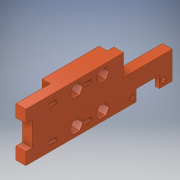
# Autodesk Inventor part: carriage Cartridge adapter
Saved by Autodesk Inventor 2018 (Build 220112000, 112)
## iProperties
Created: 2013-09-29
Part Number: carriage Cartridge adapter
Material: ABS Plastic
Document SubType Name: Modeling
Designer: Gabriel Smolnycki
Mass: 15.6927 g
Surface Area: 77.7092 cm^2
Volume: 14.8045 cm^3
Density: 1.06 g/cm^3
Appearance: Smooth - Light Orange
Author: Gabriel Smolnycki
Sending System: SolidWorks 2017
Last Author: Gabriel Smolnycki
Last Saved: 2017-09-14
Autodesk Inventor part; units mm, degrees
ref_plane "Work Plane1" through (0, 30, 0) normal (0, 1, 0) x (-1, 0, 0)
sketch "Sketch1" plane through (0, 30, 0) normal (0, 1, 0) x (-1, 0, 0)
  line L0 (-11, 41) -> (-11, -48.8)
  line L1 (0, -15) -> (-5, -15)
  line L2 (0, -15) -> (0, 41)
  line L3 (0, 41) -> (-11, 41)
  line L4 (-11, -48.8) -> (-5, -48.8)
  line L5 (-5, -48.8) -> (-5, -15)
  constraints: 12 end point, 3 horizontal, 3 vertical
extrude "Extrusion16" add sketch "Sketch1" against normal blind 30
ref_plane "Work Plane2" through (0, 0, -40.8) normal (0, 0, 1) x (1, 0, 0)
sketch "Sketch2" plane through (0, 0, -40.8) normal (0, 0, 1) x (1, 0, 0)
  line L0 (5, 7) -> (11, 7)
  line L1 (5, 0) -> (5, 7)
  line L2 (11, 0) -> (11, 7)
  line L3 (11, 0) -> (5, 0)
  constraints: 8 end point, 2 horizontal, 2 vertical
extrude "Extrusion15" cut sketch "Sketch2" along normal blind 14
sketch "Sketch3" plane through (11, 30, 41) normal (1, 0, 0) x (0, 0, -1)
  line L0 (40.5, -4) -> (35.5, -4)
  line L1 (40.5, -26) -> (40.5, -4)
  line L2 (35.5, -4) -> (35.5, -26)
  line L3 (35.5, -26) -> (40.5, -26)
  constraints: 8 end point, 2 horizontal, 2 vertical
extrude "Extrusion14" cut sketch "Sketch3" against normal blind 11
ref_plane "Work Plane3" through (0, 21, 0) normal (0, 1, 0) x (-1, 0, 0)
sketch "Sketch4" plane through (0, 21, 0) normal (0, 1, 0) x (-1, 0, 0)
  line L0 (0, 41) -> (-2, 41)
  line L1 (0, 5.5) -> (0, 41)
  line L2 (0, 5.5) -> (-2, 5.5)
  line L3 (-2, 5.5) -> (-2, 41)
  constraints: 8 end point, 2 horizontal, 2 vertical
extrude "Extrusion13" cut sketch "Sketch4" against normal blind 12
sketch "Sketch5" plane through (0, 30, 0) normal (0, 1, 0) x (-1, 0, 0)
  line L0 (-11, -48.8) -> (-11, -19)
  line L1 (-5, -19) -> (-5, -48.8)
  line L2 (-5, -19) -> (-11, -19)
  line L3 (-5, -48.8) -> (-11, -48.8)
  constraints: 8 end point, 2 horizontal, 2 vertical
extrude "Extrusion12" cut sketch "Sketch5" against normal blind 13
sketch "Sketch6" plane through (0, 21, 0) normal (0, 1, 0) x (-1, 0, 0)
  line L0 (0, -15) -> (-2, -15)
  line L1 (0, -15) -> (0, 0.5)
  line L2 (-2, 0.5) -> (0, 0.5)
  line L3 (-2, -15) -> (-2, 0.5)
  constraints: 8 end point, 2 horizontal, 2 vertical
extrude "Extrusion11" cut sketch "Sketch6" against normal blind 12
sketch "Sketch7" plane through (0, 30, 41) normal (0, 0, 1) x (1, 0, 0)
  line L0 (5, 0) -> (5, -30)
  line L1 (0, 0) -> (5, 0)
  line L2 (2, -21) -> (2, -9)
  line L3 (0, -30) -> (5, -30)
  line L4 (2, -9) -> (0, -9)
  line L5 (0, -21) -> (0, -30)
  line L6 (0, 0) -> (0, -9)
  line L7 (0, -21) -> (2, -21)
  constraints: 16 end point, 4 horizontal, 4 vertical, 2 equal length
extrude "Extrusion10" cut sketch "Sketch7" against normal blind 21
sketch "Sketch8" plane through (5, 0, 41) normal (-1, 0, 0) x (0, 0, 1)
  line L0 (-67.8, 7) -> (-81.8, 7)
  line L1 (-89.8, 0) -> (-89.8, 8)
  line L2 (-60, 8) -> (-60, 0)
  line L3 (-60, 0) -> (-67.8, 0)
  line L4 (-81.8, 7) -> (-81.8, 0)
  line L5 (-89.8, 8) -> (-60, 8)
  line L6 (-67.8, 0) -> (-67.8, 7)
  line L7 (-81.8, 0) -> (-89.8, 0)
  constraints: 16 end point, 4 horizontal, 4 vertical, 2 equal length
extrude "Extrusion9" cut sketch "Sketch8" against normal blind 3.5 draft 0
ref_plane "Work Plane4" through (0, 7.5, 0) normal (0, 1, 0) x (-1, 0, 0)
sketch "Sketch9" plane through (0, 7.5, 0) normal (0, 1, 0) x (-1, 0, 0)
  line L0 (-11, 37) -> (-5, 37)
  line L1 (-5, 41) -> (-5, 37)
  line L2 (-11, 41) -> (-11, 37)
  line L3 (-11, 41) -> (-5, 41)
  constraints: 8 end point, 2 horizontal, 2 vertical
extrude "Extrusion8" cut sketch "Sketch9" along normal blind 15 draft 0
sketch "Sketch10" plane through (11, 0, -26.8) normal (1, 0, 0) x (0, 0, -1)
  line L0 (-32.3, 24) -> (-27.3, 24)
  line L1 (-27.3, 24) -> (-27.3, 6)
  line L2 (-27.3, 6) -> (-32.3, 6)
  line L3 (-32.3, 6) -> (-32.3, 24)
  constraints: 8 end point, 2 horizontal, 2 vertical
extrude "Extrusion7" add sketch "Sketch10" against normal blind 6
sketch "Sketch11" plane through (11, 0, -26.8) normal (1, 0, 0) x (0, 0, -1)
  line L0 (-48.8, 24) -> (-48.8, 26)
  line L1 (-53.8, 24) -> (-48.8, 24)
  line L2 (-48.8, 26) -> (-53.8, 26)
  line L3 (-53.8, 26) -> (-53.8, 24)
  constraints: 8 end point, 2 horizontal, 2 vertical
extrude "Extrusion6" cut sketch "Sketch11" against normal blind 6 draft 0
sketch "Sketch12" plane through (5, 0, -26.8) normal (-1, 0, 0) x (0, 0, 1)
  line L0 (53.8, 4) -> (48.8, 4)
  line L1 (53.8, 6) -> (53.8, 4)
  line L2 (48.8, 4) -> (48.8, 6)
  line L3 (48.8, 6) -> (53.8, 6)
  constraints: 8 end point, 2 horizontal, 2 vertical
extrude "Extrusion5" cut sketch "Sketch12" against normal blind 6
sketch "Sketch13" plane through (11, 0, -26.8) normal (1, 0, 0) x (0, 0, -1)
  line L0 (-32.7585, 5.5) -> (-34.7793, 9)
  line L1 (-40.8415, 5.5) -> (-38.8207, 2)
  line L2 (-38.8207, 2) -> (-34.7793, 2)
  line L3 (-34.7793, 9) -> (-38.8207, 9)
  line L4 (-34.7793, 2) -> (-32.7585, 5.5)
  line L5 (-38.8207, 9) -> (-40.8415, 5.5)
  constraints: 12 end point, 5 equal length, 2 horizontal
extrude "Extrusion4" cut sketch "Sketch13" against normal blind 6
sketch "Sketch14" plane through (11, 0, -26.8) normal (1, 0, 0) x (0, 0, -1)
  line L0 (-34.7793, 21) -> (-32.7585, 24.5)
  line L1 (-38.8207, 28) -> (-40.8415, 24.5)
  line L2 (-32.7585, 24.5) -> (-34.7793, 28)
  line L3 (-40.8415, 24.5) -> (-38.8207, 21)
  line L4 (-38.8207, 21) -> (-34.7793, 21)
  line L5 (-34.7793, 28) -> (-38.8207, 28)
  constraints: 12 end point, 5 equal length, 2 horizontal
extrude "Extrusion3" cut sketch "Sketch14" against normal blind 6
sketch "Sketch15" plane through (11, 0, -26.8) normal (1, 0, 0) x (0, 0, -1)
  line L0 (-18.7793, 21) -> (-16.7585, 24.5)
  line L1 (-22.8207, 28) -> (-24.8415, 24.5)
  line L2 (-16.7585, 24.5) -> (-18.7793, 28)
  line L3 (-24.8415, 24.5) -> (-22.8207, 21)
  line L4 (-22.8207, 21) -> (-18.7793, 21)
  line L5 (-18.7793, 28) -> (-22.8207, 28)
  constraints: 12 end point, 5 equal length, 2 horizontal
extrude "Extrusion2" cut sketch "Sketch15" against normal blind 6 draft 0
sketch "Sketch16" plane through (11, 0, -26.8) normal (1, 0, 0) x (0, 0, -1)
  line L0 (-18.7793, 2) -> (-16.7585, 5.5)
  line L1 (-22.8207, 9) -> (-24.8415, 5.5)
  line L2 (-16.7585, 5.5) -> (-18.7793, 9)
  line L3 (-24.8415, 5.5) -> (-22.8207, 2)
  line L4 (-22.8207, 2) -> (-18.7793, 2)
  line L5 (-18.7793, 9) -> (-22.8207, 9)
  constraints: 12 end point, 5 equal length, 2 horizontal
extrude "Extrusion1" cut sketch "Sketch16" against normal blind 6 draft 0
hole "Hole6" at (11, 3.5, -24.1) direction (-1, 0, 0) diameter 3.2 depth 2.5
hole "Hole5" at (11, 3.5, -43.1) direction (-1, 0, 0) diameter 3.2 depth 2.5
hole "Hole4" at (0, 24.5, 10) direction (1, 0, 0) diameter 4.2 depth 5
sketch "Sketch19" plane through (0, 0, 0) normal (1, 0, 0) x (0, 1, 0)
  point P0 (24.5, 10)
hole "Hole3" at (0, 5.5, 10) direction (1, 0, 0) diameter 4.2 depth 5
sketch "Sketch18" plane through (11, 0, -26.8) normal (1, 0, 0) x (0, 0, -1)
  point P0 (16.3, 3.5)
hole "Hole2" at (0, 24.5, -6) direction (1, 0, 0) diameter 4.2 depth 5
sketch "Sketch17" plane through (11, 0, -26.8) normal (1, 0, 0) x (0, 0, -1)
  point P0 (-2.7, 3.5)
hole "Hole1" at (0, 5.5, -6) direction (1, 0, 0) diameter 4.2 depth 5
sketch "Sketch20" plane through (0, 0, 0) normal (1, 0, 0) x (0, 1, 0)
  point P0 (5.5, 10)
sketch "Sketch21" plane through (0, 0, 0) normal (1, 0, 0) x (0, 1, 0)
  point P0 (24.5, -6)
sketch "Sketch22" plane through (0, 0, 0) normal (1, 0, 0) x (0, 1, 0)
  point P0 (5.5, -6)
body "Solid3"
